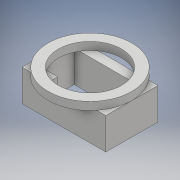
# Autodesk Inventor part: baseRotor1
Saved by Autodesk Inventor 2017 (Build 210142000, 142)
## iProperties
Created: 2017-08-06
Part Number: baseRotor1
Material: Generic
Document SubType Name: Sheet Metal
Designer: Bardo91
Density: 1 g/cm^3
Sheet Metal Rule: Default_mm
Appearance: Default
Author: Bardo91
Autodesk Inventor part; units mm, degrees
ref_plane "YZ Plane" through (0, 0, 0) normal (1, 0, 0) x (0, 1, 0)
ref_plane "XZ Plane" through (0, 0, 0) normal (0, 1, 0) x (-1, 0, 0)
ref_plane "XY Plane" through (0, 0, 0) normal (0, 0, 1) x (1, 0, 0)
sketch "Sketch8" plane through (0, 0, 0) normal (0, 0, 1) x (1, 0, 0)
  line L0 (0, 0) -> (41, 0)
  line L1 (41, 0) -> (41, 21)
  line L2 (41, 21) -> (0, 21)
  line L3 (0, 21) -> (0, 0)
  line L4 (-6, 27) -> (47, 27)
  line L5 (47, 27) -> (47, -6)
  line L6 (47, -6) -> (-6, -6)
  line L7 (-6, -6) -> (-6, 27)
  dimension "d35" = 41
  dimension "d36" = 21
  dimension "d37" = 6
  constraints: 16 end point, 6 perpendicular, 1 horizontal, 3 other
  measures "d35" distance of L0.start L0.end
  measures "d36" distance of L0.end L1.end
  measures "d37" distance between parallel lines of L2 L4
extrude "Extrusion8" add sketch "Sketch8" along normal blind 20
sketch "Sketch9" plane through (0, 0, 20) normal (0, 0, 1) x (1, 0, 0)
  line L0 (41, 0) -> (0, 0) projected
  line L1 (20.5, 0) -> (10.5, 0)
  line L2 (10.5, 0) -> (10.5, -5)
  line L3 (10.5, -5) -> (30.5, -5)
  line L4 (30.5, -5) -> (30.5, 0)
  line L5 (30.5, 0) -> (20.5, 0)
  dimension "d45" = 10
  dimension "d46" = 5
  dimension "d47" = 20
  dimension "d48" = 5
  constraints: 10 end point, 2 perpendicular, 2 point on line, 1 collinear, 1 midpoint
  measures "d45" distance of L1.start L1.end
  measures "d46" distance of L1.end L2.end
  measures "d47" distance of L2.end L3.end
  measures "d48" distance of L3.end L4.end
extrude "Extrusion9" cut sketch "Sketch9" against normal up to next
sketch "Sketch10" plane through (0, 0, 20) normal (0, 0, 1) x (1, 0, 0)
  line L0 (0, 21) -> (0, 0) projected
  line L1 (0, 10.5) -> (41, 10.5)
  line L2 (41, 21) -> (41, 0) projected
  circle A0 centre (20.5, 10.5) radius 20
  circle A1 centre (20.5, 10.5) radius 26.5
  line L3 (47, 27) -> (47, -6) projected
  dimension "d51" = 40
  constraints: 3 midpoint, 2 centre point, 2 end point, 1 coincident, 1 tangent
  measures "d51" diameter of A0
extrude "Extrusion10" add sketch "Sketch10" along normal blind 5
equation "\"BendRadius\" = Thickness"
equation "\"BendReliefWidth\" = Thickness"
equation "\"BendReliefDepth\" = 0.5 * Thickness"
equation "\"CornerReliefSize\" = 4 * Thickness"
equation "\"MinimumRemnant\" = 2 * Thickness"
equation "\"TransitionRadius\" = BendRadius"
equation "\"JacobiRadiusSize\" = BendRadius"
equation "\"GapSize\" = Thickness"
equation "\"Thickness\" = 0.5"
body "Solid2"
